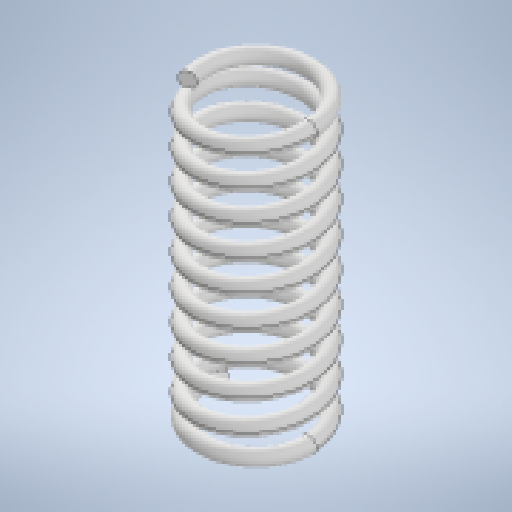
# Autodesk Inventor part: Sprint
Saved by Autodesk Inventor 2023 (Build 270158000, 158)
## iProperties
Created: 2023-05-05
Part Number: Sprint
Material: Generic
Document SubType Name: Modeling
Designer: Nathann
Density: 1 g/cm^3
Appearance: Default
Author: Nathann
Autodesk Inventor part; units mm, degrees
ref_plane "YZ Plane" through (0, 0, 0) normal (1, 0, 0) x (0, 1, 0)
ref_plane "XZ Plane" through (0, 0, 0) normal (0, 1, 0) x (-1, 0, 0)
ref_plane "XY Plane" through (0, 0, 0) normal (0, 0, 1) x (1, 0, 0)
sketch "Sketch1" plane through (0, 0, 0) normal (0, 0, 1) x (1, 0, 0)
  circle A0 centre (0, 0) radius 0.5
  line L0 (-3.5, 0) -> (-3.5, 42.2657)
  dimension "d0" = 1
  dimension "d1" = 3.5
  constraints: 2 end point, 1 centre point, 1 coincident, 1 vertical
  measures "d0" diameter of A0
  measures "d1" distance from line of point (0, 0) L0
coil "Coil1" sketch "Sketch1" operation add axis through (-3.5, 0, 0) along (0, 1, 0) pitch 2 turns 9 hand right
sketch "Sketch2" plane through (0, 18, 0) normal (0, 0, -1) x (-1, 0, 0)
  circle A0 centre (0, 0) radius 0.5
  line L0 (3.5, 0) -> (3.5, 1.0848)
  point P0 (0, -18)
  point P1 (-0.5, 0)
  point P2 (3.5, 0.5424)
  dimension "d10" = 3.5
  constraints: 2 end point, 1 horizontal alignment, 1 midpoint, 1 vertical, 2 other
  measures "d10" horizontal distance of point (0, 0) point (3.5, 0.542)
revolve "Revolution1" add sketch "Sketch2" angle 200 about axis through (-3.5, 18, 0) along (0, 1, 0)
sketch "Sketch3" plane through (0, 0, 0) normal (0, 0, 1) x (1, 0, 0)
  circle A0 centre (0, 0) radius 0.5 projected
  line L0 (-3.5, 0) -> (-3.5, -1.871)
  point P0 (0.5, 0)
  dimension "d12" = 3.5
  constraints: 2 end point, 1 horizontal alignment, 1 vertical
  measures "d12" distance from line of point (0, 0) L0
revolve "Revolution2" add sketch "Sketch3" angle 200 about axis through (-3.5, 0, 0) along (0, -1, 0)
body "Solid1"
